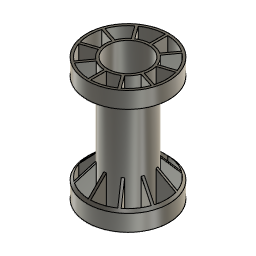
Part Demo (Autodesk Fusion 360 design; units mm, degrees)
Autodesk Fusion 360 part; units mm, degrees
sketch "Sketch1" plane through (0, 0, 0) normal (1, 0, 0) x (0, 1, 0)
  line L0 (25, 0) -> (25, 150)
  line L1 (25, 150) -> (50, 150)
  line L2 (50, 150) -> (50, 130)
  line L3 (50, 130) -> (28, 130)
  line L4 (28, 130) -> (28, 42)
  line L5 (28, 42) -> (50, 20)
  line L6 (50, 20) -> (50, 0)
  line L7 (50, 0) -> (25, 0)
  line L8 (0, 0) -> (0, 146.3043) construction
  dimension "d1" = 3
  dimension "d2" = 25
  dimension "d3" = 150
  dimension "d4" = 50
  dimension "d5" = 20
  dimension "d6" = 20
  dimension "d7" = 135
  constraint vertical L0
  constraint perpendicular L0 L1
  constraint perpendicular L1 L2
  constraint perpendicular L2 L3
  constraint perpendicular L1 L4
  constraint parallel L4 L6
  constraint horizontal L7
  constraint coincident L8.start L7
  constraint collinear L2 L6
  constraint coincident L8.start origin
  constraint parallel L0 L8
  measures "d1" distance of L0 L4
  measures "d2" distance of L8.start L0
  measures "d3" distance of L0.start L0.end
  measures "d4" distance of L8.start L6
  measures "d5" distance of L5.end L6.end
  measures "d6" distance of L1.end L2.end
  measures "d7" angle of L5 L6
revolve "Revolve1" add sketch "Sketch1" angle 360 about axis through (0, 0, 0) along (0, 0, 1)
sketch "Sketch2" plane through (0, 0, 150) normal (0, 0, 1) x (-1, 0, 0)
  circle A0 centre (0, 0) radius 25
  circle A1 centre (0, 0) radius 50
  line L0 (0, 0) -> (-29.3893, 40.4508) construction
  line L1 (0, 0) -> (0, 50) construction
  arc A2 (-1.5, 27.9598) -> (-15.2208, 23.5016) centre (0, 0) ccw
  arc A3 (-1.5, 46.9761) -> (-26.3983, 38.8861) centre (0, 0) ccw
  line L2 (-1.5, 27.9598) -> (-1.5, 46.9761)
  line L3 (-15.2208, 23.5016) -> (-26.3983, 38.8861)
  dimension "d9" = 36
  dimension "d10" = 1.5
  dimension "d11" = 1.5
  dimension "d12" = 3
  dimension "d13" = 3
  constraint coincident A0.centre A1.centre
  constraint coincident A1 L0.end
  constraint coincident A1 L1.end
  constraint vertical L1
  constraint parallel L0 L3
  constraint parallel L1 L2
  measures "d9" angle of L0 L1
  measures "d10" distance of L1 L2
  measures "d11" distance of L0 L3
  measures "d12" distance of A0 A2
  measures "d13" distance of A1 A3
extrude "Extrude1" cut sketch "Sketch2" against normal up to surface (150 mm away) contours A2 A3 L2 L3
pattern_circular "C-Pattern1" count 10 over 360 about axis through (0, 0, 150) along (0, 0, -1) of "Extrude1"
